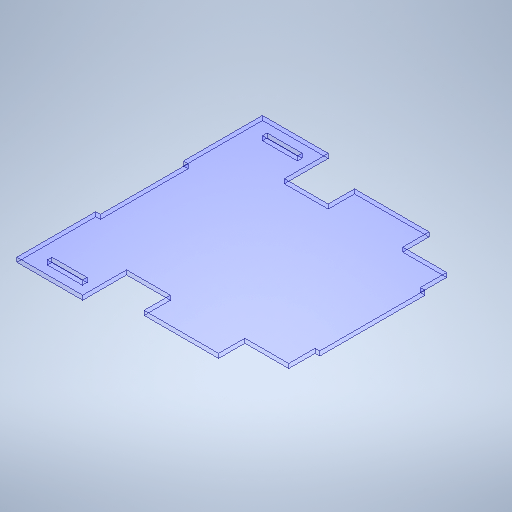
# Autodesk Inventor part: hood
Saved by Autodesk Inventor 2025.3 (Build 293356030, 356C)
## iProperties
Created: 2026-06-26
Part Number: hood
Material: Generic
Document SubType Name: Modeling
Designer: user
Density: 1 g/cm^3
Appearance: Blue
Author: user
Autodesk Inventor part; units mm, degrees
ref_plane "YZ Plane" through (0, 0, 0) normal (1, 0, 0) x (0, 1, 0)
ref_plane "XZ Plane" through (0, 0, 0) normal (0, 1, 0) x (-1, 0, 0)
ref_plane "XY Plane" through (0, 0, 0) normal (0, 0, 1) x (1, 0, 0)
sketch "Sketch1" plane through (0, 0, 0) normal (0, 1, 0) x (-1, 0, 0)
  line L0 (0, 0) -> (-75, 0)
  line L1 (-75, 0) -> (-75, -280)
  line L2 (-75, -280) -> (0, -280)
  line L3 (0, -280) -> (0, 0)
  line L4 (-20, -14.7) -> (-60, -14.7)
  line L5 (-60, -14.7) -> (-60, -20)
  line L6 (-60, -20) -> (-20, -20)
  line L7 (-20, -20) -> (-20, -14.7)
  line L8 (-75, -140) -> (0, -140) construction
  line L9 (-20, -265.3) -> (-60, -265.3)
  line L10 (-60, -265.3) -> (-60, -260)
  line L11 (-60, -260) -> (-20, -260)
  line L12 (-20, -260) -> (-20, -265.3)
  line L13 (-75, -50) -> (-260, -50)
  line L14 (-260, -50) -> (-260, -230)
  line L15 (-260, -230) -> (-75, -230)
  line L16 (-75, -230) -> (-75, -50)
  line L17 (-260, -80) -> (-265.3, -80)
  line L18 (-265.3, -80) -> (-265.3, -200)
  line L19 (-265.3, -200) -> (-260, -200)
  line L20 (-260, -200) -> (-260, -80)
  line L21 (0, -90) -> (-5.3, -90)
  line L22 (-5.3, -90) -> (-5.3, -190)
  line L23 (-5.3, -190) -> (0, -190)
  line L24 (0, -190) -> (0, -90)
  line L25 (-125, -50) -> (-210, -50)
  line L26 (-210, -50) -> (-210, -20)
  line L27 (-210, -20) -> (-125, -20)
  line L28 (-125, -20) -> (-125, -50)
  line L29 (-125, -230) -> (-210, -230)
  line L30 (-210, -230) -> (-210, -260)
  line L31 (-210, -260) -> (-125, -260)
  line L32 (-125, -260) -> (-125, -230)
  point P0 (-75, -230)
  point P1 (0, -190)
  dimension "d0" = 75
  dimension "d1" = 280
  dimension "d2" = 40
  dimension "d3" = 5.3
  dimension "d6" = 185
  dimension "d7" = 180
  dimension "d8" = 5.3
  dimension "d9" = 120
  dimension "d11" = 20
  dimension "d12" = 5.3
  dimension "d13" = 100
  dimension "d14" = 90
  dimension "d15" = 85
  dimension "d16" = 50
  constraints: 66 end point, 14 parallel, 7 horizontal, 7 perpendicular, 5 point on line, 4 symmetric about line, 2 midpoint
  measures "d0" distance of L2.end L1.end
  measures "d1" distance of L1.end L0.end
  measures "d2" distance of L6.end L5.end
  measures "d3" distance of L5.end L4.end
  measures "d6" distance of L15.end L14.end
  measures "d7" distance of L14.end L13.end
  measures "d8" distance of L19.end L18.end
  measures "d9" distance of L18.end L17.end
  measures "d11" distance between parallel lines of L12 L3
  measures "d12" distance of L23.end L22.end
  measures "d13" distance of L22.end L21.end
  measures "d14" distance of L2.end L23.end
  measures "d15" distance of L26.end L27.end
  measures "d16" distance between parallel lines of L28 L1
extrude "Extrusion1" add sketch "Sketch1" along normal blind 5 contours L3 L21 L22 L23 L2 L1 L0 | L1 L15 L14 L13 | L13 L26 L27 L28 | L32 L31 L30 L15 | L14 L19 L18 L17
body "Solid1"
